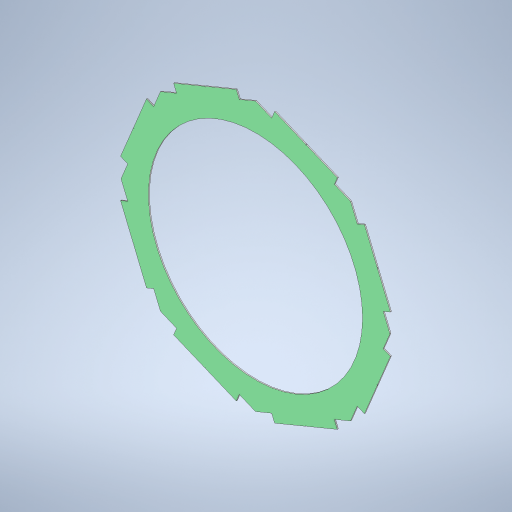
# Autodesk Inventor part: ДМФ 01 29 Барабан сборочный лист
Saved by Autodesk Inventor 2024.2 (Build 282272000, 272)
## iProperties
Created: 2024-04-28
Part Number: ДМФ 01 29 Барабан сборочный лист
Material: Generic
Document SubType Name: Sheet Metal
Designer: admin
Density: 1 g/cm^3
Flat Pattern Width: 50.9 cm
Flat Pattern Length: 50.9 cm
Flat Pattern Area: 2590.81 cm^2
Sheet Metal Rule: Default
Sheet Metal Width: 509,000 mm
Sheet Metal Length: 509,000 mm
Sheet Metal Area: 259081,000 mm^2
Appearance: Default
Stock Number: Барабан_Сборочный_Лист
Author: pokla
Autodesk Inventor part; units mm, degrees
ref_plane "YZ Plane" through (0, 0, 0) normal (1, 0, 0) x (0, 1, 0)
ref_plane "XZ Plane" through (0, 0, 0) normal (0, 1, 0) x (-1, 0, 0)
ref_plane "XY Plane" through (0, 0, 0) normal (0, 0, 1) x (1, 0, 0)
sketch "Sketch2" plane through (0, 0, 0) normal (0, 0, 1) x (1, 0, 0)
  line L0 (-194.7859, 194.7859) -> (0, 275.4688)
  line L1 (0, 275.4688) -> (194.7859, 194.7859)
  line L2 (194.7859, 194.7859) -> (275.4688, 0)
  line L3 (275.4688, 0) -> (194.7859, -194.7859)
  line L4 (194.7859, -194.7859) -> (0, -275.4688)
  line L5 (0, -275.4688) -> (-194.7859, -194.7859)
  line L6 (-194.7859, -194.7859) -> (-275.4688, 0)
  line L7 (-275.4688, 0) -> (-194.7859, 194.7859)
  circle A0 centre (0, 0) radius 206.5
  dimension "d23" = 509
  dimension "d26" = 413
  measures "d23" distance between parallel lines of L6 L2
  measures "d26" diameter of A0
extrude "Plate1" add sketch "Sketch2" against normal blind 2
sketch "Sketch5" plane through (0, 0, 0) normal (0, 0, 1) x (1, 0, 0)
  line L0 (0, -275.4688) -> (194.7859, -194.7859) projected
  line L1 (98.3168, -234.7447) -> (97.0103, -234.2035)
  line L2 (97.0103, -234.2035) -> (96.4691, -235.51)
  line L3 (97.0103, -234.2035) -> (97.3929, -235.1273) construction
  point P0 (0, 0)
  dimension "d30" = 1
  constraints: 6 end point, 3 perpendicular, 2 point on line, 1 midpoint
  measures "d30" distance of L1.end L3.end
extrude "Extrusion2" cut sketch "Sketch5" along normal through all both and the other way through all
pattern_circular "Circular Pattern2" count 8 over 360 about axis through (0, 0, -10) along (0, 0, 1) of "Extrusion2"
sketch "Sketch6" plane through (0, 0, 0) normal (0, 0, 1) x (1, 0, 0)
  line L0 (0, 275.4688) -> (-96.4691, 235.51) projected
  line L1 (96.4691, 235.51) -> (0, 275.4688) projected
  line L2 (0, 275.4688) -> (-36.9552, 260.1615)
  line L3 (0, 275.4688) -> (36.9552, 260.1615)
  line L4 (-31.2149, 246.3033) -> (0, 259.2329)
  line L5 (0, 259.2329) -> (31.2149, 246.3033)
  line L6 (31.2149, 246.3033) -> (36.9552, 260.1615)
  line L7 (-31.2149, 246.3033) -> (-36.9552, 260.1615)
  point P0 (0, 0)
  dimension "d36" = 40
  dimension "d37" = 15
  constraints: 12 end point, 2 perpendicular, 2 point on line, 1 equal length, 1 other
  measures "d36" distance of L2.end L0.start
  measures "d37" distance between parallel lines of L2 L4
extrude "Extrusion3" cut sketch "Sketch6" against normal through all
pattern_circular "Circular Pattern3" count 8 over 360 about axis through (0, 0, 0) along (0, 0, -1) of "Extrusion3"
equation "\"d23\" = Барабан_габарит_по_кассетам - 2 * Thickness"
equation "\"d15\" = Thickness"
equation "\"BendRadius\" = Thickness"
equation "\"BendReliefWidth\" = Thickness"
equation "\"BendReliefDepth\" = 0.5 * Thickness"
equation "\"CornerReliefSize\" = 4 * Thickness"
equation "\"MinimumRemnant\" = 2 * Thickness"
equation "\"TransitionRadius\" = BendRadius"
equation "\"JacobiRadiusSize\" = BendRadius"
equation "\"GapSize\" = Thickness"
equation "\"Барабан_габарит_по_кассетам\" = 513"
equation "\"Thickness\" = 2"
body "Solid1"
